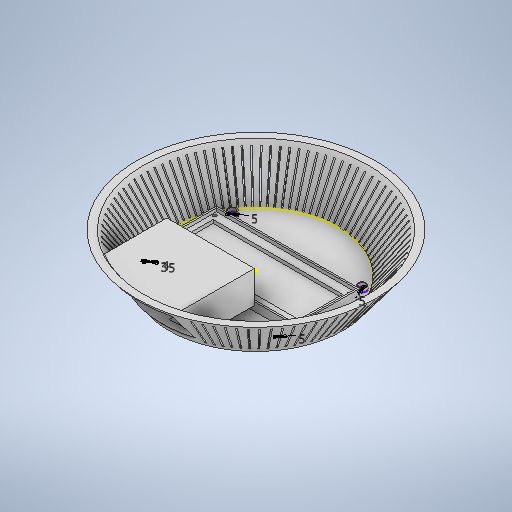
# Autodesk Inventor part: Base
Saved by Autodesk Inventor 2025.2 (Build 292293000, 293)
## iProperties
Created: 2026-03-13
Part Number: Base
Material: Genérico
Document SubType Name: Modeling
Designer: Periscopio
Density: 1 g/cm^3
Appearance: Valor por defecto
Author: Periscopio
Autodesk Inventor part; units mm, degrees
note: some values were not read from the file. Chosen so that the rebuilt part matches the saved one: direction of "Repujado1".
ref_plane "YZ Plane" through (0, 0, 0) normal (1, 0, 0) x (0, 1, 0)
ref_plane "XZ Plane" through (0, 0, 0) normal (0, 1, 0) x (-1, 0, 0)
sketch "Boceto1" plane through (0, 0, 0) normal (0, 0, 1) x (1, 0, 0)
  line L0 (0, 0) -> (51, 0)
  line L1 (51, 0) -> (71, 27)
  line L2 (71, 27) -> (0, 27)
  line L3 (0, 27) -> (0, 0)
  dimension "d1" = 71
  dimension "d2" = 27
  dimension "d3" = 51
  constraints: 8 end point, 1 horizontal, 1 parallel, 1 perpendicular
  measures "d1" distance of L1.end L2.end
  measures "d2" distance of L2.end L0.start
  measures "d3" distance of L0.start L0.end
revolve "Revolución1" add sketch "Boceto1" angle 360 about axis through (0, 27, 0) along (0, -1, 0)
shell "Vaciado2" thickness 3.5 removed faces 1 at (22.3843, 27, 7.6846)
sketch "Boceto3" plane through (0, 3.5, 0) normal (0, 1, 0) x (1, 0, 0)
  line L0 (41.5, 18) -> (-41.5, 18)
  line L1 (-41.5, 18) -> (-41.5, -18)
  line L2 (-41.5, -18) -> (41.5, -18)
  line L3 (41.5, -18) -> (41.5, 18)
  line L4 (-42.5, -19) -> (42.5, -19)
  line L5 (42.5, -19) -> (42.5, 19)
  line L6 (42.5, 19) -> (-42.5, 19)
  line L7 (-42.5, 19) -> (-42.5, -19)
  line L8 (-42.5, -19) -> (42.5, 19) construction
  line L9 (42.5, -19) -> (-42.5, 19) construction
  line L10 (-38.5, -13) -> (38.5, -13)
  line L11 (38.5, -13) -> (38.5, 13)
  line L12 (38.5, 13) -> (-38.5, 13)
  line L13 (-38.5, 13) -> (-38.5, -13)
  line L14 (-38.5, -13) -> (38.5, 13) construction
  line L15 (38.5, -13) -> (-38.5, 13) construction
  point P0 (0, 0)
  dimension "d22" = 83
  dimension "d26" = 85
  dimension "d27" = 38
  dimension "d28" = 77
  dimension "d29" = 26
  dimension "d34" = 1
  dimension "d35" = 1
  dimension "d36" = 1
  dimension "d37" = 1
  dimension "d51" = 36
  constraints: 32 end point, 7 parallel, 4 midpoint, 3 horizontal, 3 perpendicular
  measures "d22" distance of L0.start L0.end
  measures "d26" distance of L6.end L5.end
  measures "d27" distance of L5.end L4.end
  measures "d28" distance of L12.end L11.end
  measures "d29" distance of L11.end L10.end
  measures "d34" distance between parallel lines of L6 L0
  measures "d35" distance between parallel lines of L4 L2
  measures "d36" distance between parallel lines of L5 L3
  measures "d37" distance between parallel lines of L7 L1
  measures "d51" distance of L2.end L0.start
extrude "Extrusión1" add sketch "Boceto3" along normal blind 1 contours L3 L2 L1 L0 | L13 L12 L11 L10
extrude "Extrusión2" add sketch "Boceto3" along normal blind 5 contours L7 L6 L5 L4
extrude "Extrusión3" add sketch "Boceto3" along normal blind 3 contours L3 L2 L1 L0
sketch "Boceto6" plane through (0, 6.5, 0) normal (0, 1, 0) x (1, 0, 0)
  point P0 (0, 0)
sketch "Boceto8" plane through (-42.5, 3.5, 19) normal (0, 0, 1) x (1, 0, 0)
  line L0 (84, 3) -> (1, 3) projected
  line L1 (84, 5) -> (1, 5) projected
  line L2 (85, 0) -> (0, 0) projected
  line L3 (42.5, 0) -> (42.5, 5)
  line L4 (42.5, 0) -> (78.5811, 0)
  line L5 (78.5811, 0) -> (7.5, 0)
  line L6 (18.0405, 0) -> (68.0405, 0)
  line L7 (16.4402, -0.1344) -> (66.3733, 21.024) construction
  line L8 (66.4399, 0.0241) -> (16.3736, 20.8654) construction
  line L9 (15.4433, -1.1376) -> (67.3702, 22.0271) construction
  line L10 (67.5055, -1.0002) -> (15.308, 21.8897) construction
  line L11 (15.4433, -1.1376) -> (16.4433, -1.1376)
  line L12 (66.5055, -1.0002) -> (67.5055, -1.0002)
  line L13 (60.4951, 3.0767) -> (60.4951, 2.0741)
  line L14 (60.4951, 2.0741) -> (8.4951, 2.0741)
  line L15 (8.4951, 2.0741) -> (8.4951, 22.0741)
  line L16 (8.4951, 22.0741) -> (60.4951, 22.0741)
  line L17 (60.4951, 22.0741) -> (60.4951, 2.0741)
  line L18 (59.4951, 3.0741) -> (9.4951, 3.0741)
  line L19 (9.4951, 3.0741) -> (9.4951, 21.0741)
  line L20 (9.4951, 21.0741) -> (59.4951, 21.0741)
  line L21 (59.4951, 21.0741) -> (59.4951, 3.0741)
  point P0 (42.5, -3.5)
  point P1 (41.4067, 10.4448)
  point P2 (42.5, 3)
  point P3 (60.4951, 3)
  point P4 (42.5, 2.0741)
  dimension "d69" = 52
  dimension "d70" = 20
  dimension "d71" = 50
  dimension "d72" = 18
  dimension "d73" = 1
  dimension "d74" = 1
  constraints: 38 end point, 7 horizontal, 6 midpoint, 4 parallel, 3 perpendicular, 2 point on line, 1 vertical
  measures "d69" distance of L15.end L16.end
  measures "d70" distance of L14.end L15.end
  measures "d71" distance of L19.end L20.end
  measures "d72" distance of L18.end L19.end
  measures "d73" distance between parallel lines of L17 L21
  measures "d74" distance between parallel lines of L14 L18
extrude "Extrusión5" cut sketch "Boceto8" along normal blind 55 contours L18 L19 L1 L3 | L3 L1 L21 L18 | L1 L19 L20 L21
extrude "Extrusión7" add sketch "Boceto8" along normal up to next contours L0 L3 L18 L21 L1 L17 L13 | L3 L14 L15 L0 | L0 L15 L1 L19 L18 L3 | L1 L21 L20 L19 L15 L16 L17
sketch "Boceto9" plane through (-33.0049, 6.5741, 19) normal (0, 0, 1) x (1, 0, 0)
  line L0 (50, 18) -> (0, 18) projected
  line L1 (0, 0) -> (50, 0) projected
  line L2 (0, 18) -> (50, 18)
  line L3 (50, 18) -> (50, 0)
  line L4 (50, 0) -> (0, 0)
  line L5 (0, 0) -> (0, 18)
  line L6 (5.0356, 17.9033) -> (25.0356, 17.9033)
  line L7 (25.0356, 17.9033) -> (25.0356, 1.9033)
  line L8 (25.0356, 1.9033) -> (5.0356, 1.9033)
  line L9 (5.0356, 1.9033) -> (5.0356, 17.9033)
  circle A0 centre (39.3418, 9.9033) radius 2.5
  point P0 (33.0049, -6.5741)
  dimension "d75" = 20
  dimension "d76" = 16
  dimension "d77" = 5
  constraints: 16 end point, 4 parallel, 2 horizontal, 2 perpendicular, 1 centre point
  measures "d75" distance of L7.end L8.end
  measures "d76" distance of L6.end L7.end
  measures "d77" diameter of A0
extrude "Extrusión8" add sketch "Boceto9" along normal blind 2
sketch "Boceto10" plane through (0, 6.5, 0) normal (0, 1, 0) x (1, 0, 0)
  line L0 (38.5, 13) -> (-38.5, 13) projected
  line L1 (-41.5, -18) -> (-41.5, 18) projected
  circle A0 centre (-40, 15.5) radius 1
  circle A1 centre (-40, -15.5) radius 1
  circle A2 centre (40, 15.5) radius 1
  circle A3 centre (40, -15.5) radius 1
  point P0 (0, 0)
  dimension "d80" = 2
  dimension "d83" = 31
  dimension "d86" = 80
  constraints: 4 centre point, 1 horizontal, 1 vertical, 6 other
  measures "d80" diameter of A0
  measures "d83" distance of A0.centre A1.centre
  measures "d86" distance of A0.centre A2.centre
extrude "Extrusión9" cut sketch "Boceto10" against normal blind 4
thread "Rosca1" size "M2x0.4" class "6H" standard "ANSI Metric M Profile" full length
thread "Rosca2" size "M2x0.4" class "6H" standard "ANSI Metric M Profile" full length
thread "Rosca3" size "M2x0.4" class "6H" standard "ANSI Metric M Profile" full length
thread "Rosca4" size "M2x0.4" class "6H" standard "ANSI Metric M Profile" full length
fillet "Empalme1" radius 2 1 edges at (-51, 0, 0)
sketch "Boceto11" plane through (0, 3.5, 0) normal (0, 1, 0) x (1, 0, 0)
  circle A0 centre (-38.5311, -24.4651) radius 1.5
  circle A1 centre (-38.5311, -24.4651) radius 2
  line L0 (-42.5, 19) -> (42.5, 19) projected
  circle A2 centre (0, 0) radius 49.237 projected
  circle A3 centre (-38.5311, 24.4651) radius 1.5
  circle A4 centre (-38.5311, 24.4651) radius 2
  circle A5 centre (38.5311, -24.4651) radius 1.5
  circle A6 centre (38.5311, -24.4651) radius 2
  circle A7 centre (38.5311, 24.4651) radius 2
  circle A8 centre (38.5311, 24.4651) radius 1.5
  circle A9 centre (-38.5311, 24.4651) radius 2.5
  circle A10 centre (38.5311, 24.4651) radius 2.5
  circle A11 centre (38.5311, -24.4651) radius 2.5
  circle A12 centre (-38.5311, -24.4651) radius 2.5
  point P0 (0, 0)
  dimension "d100" = 3
  dimension "d101" = 4
  dimension "d107" = 5
  dimension "d108" = 5
  dimension "d109" = 5
  dimension "d110" = 5
  constraints: 12 centre point, 8 coincident
  measures "d100" diameter of A0
  measures "d101" diameter of A1
  measures "d107" diameter of A9
  measures "d108" diameter of A10
  measures "d109" diameter of A11
  measures "d110" diameter of A12
extrude "Extrusión10" cut sketch "Boceto11" against normal up to next contours A0 | A3 | A5 | A8
extrude "Extrusión11" add sketch "Boceto11" along normal blind 2 contours A9 | A10 | A11 | A12
ref_plane "Plano de trabajo3" through (0, 0, -71.75) normal (0, 0, 1) x (1, 0, 0)
sketch "Boceto14" plane through (0, 0, -71.75) normal (0, 0, 1) x (1, 0, 0)
  line L0 (-33.0049, 24.5741) -> (16.9951, 24.5741) projected
  line L1 (0.4, 3.6364) -> (-0.4, 3.6364)
  line L2 (-0.4, 3.6364) -> (-0.4, 24.5741)
  line L3 (-0.4, 24.5741) -> (0.4, 24.5741)
  line L4 (0.4, 24.5741) -> (0.4, 3.6364)
  line L5 (0.4, 3.6364) -> (-0.4, 24.5741) construction
  line L6 (-0.4, 3.6364) -> (0.4, 24.5741) construction
  line L7 (0, 6.5) -> (0, 5.5741) projected
  point P0 (0, 0)
  point P1 (0, 14.1052)
  dimension "d129" = 0.8
  dimension "d130" = 0.4
  constraints: 12 end point, 2 midpoint, 2 parallel, 1 horizontal, 1 perpendicular, 1 point on line
  measures "d129" distance of L1.start L1.end
  measures "d130" distance between parallel lines of L7 L4
emboss "Repujado1" sketch "Boceto14" operation cut depth 4 direction (0, 0, 1)
pattern_circular "Patrón circular1" count 40 over 140 about axis through (0, -10, 0) along (0, 1, 0) of "Repujado1"
pattern_circular "Patrón circular2" count 40 over 158 about axis through (0, -10, 0) along (0, -1, 0) of "Repujado1"
